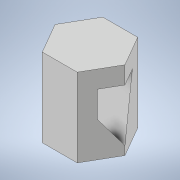
# Autodesk Inventor part: Деталь1
Saved by Autodesk Inventor 2021.2 (Build 252289000, 289)
## iProperties
Created: 2023-10-05
Part Number: Деталь1
Material: Типовые
Document SubType Name: Modeling
Designer: User
Density: 1 g/cm^3
Appearance: По умолчанию
Author: User
Autodesk Inventor part; units mm, degrees
ref_plane "YZ Plane" through (0, 0, 0) normal (1, 0, 0) x (0, 1, 0)
ref_plane "XZ Plane" through (0, 0, 0) normal (0, 1, 0) x (-1, 0, 0)
ref_plane "XY Plane" through (0, 0, 0) normal (0, 0, 1) x (1, 0, 0)
sketch "Эскиз1" plane through (0, 0, 0) normal (0, 1, 0) x (-1, 0, 0)
  circle A0 centre (0, 0) radius 40
  line L0 (40, 0) -> (20, -34.641)
  line L1 (20, -34.641) -> (-20, -34.641)
  line L2 (-20, -34.641) -> (-40, 0)
  line L3 (-40, 0) -> (-20, 34.641)
  line L4 (-20, 34.641) -> (20, 34.641)
  line L5 (20, 34.641) -> (40, 0)
  dimension "d0" = 80
  constraints: 12 end point, 2 coincident, 1 horizontal alignment, 15 other
extrude "Выдавливание1" add sketch "Эскиз1" along normal blind 90 contours L0 L1 L2 L3 L4 L5
sketch "Эскиз3" plane through (0, 0, 0) normal (1, 0, 0) x (0, 1, 0)
  line L0 (0, 0) -> (10, 0)
  line L1 (90, 0) -> (70, 0)
  line L2 (70, 0) -> (70, -20)
  line L3 (70, -20) -> (10, 0)
  line L4 (70, 0) -> (70, 20)
  line L5 (70, 20) -> (40, 20)
  line L6 (40, 20) -> (10, 0)
  constraints: 14 end point, 3 perpendicular
extrude "Выдавливание3" cut sketch "Эскиз3" against normal mid plane 90
